Autodesk Inventor part; units mm, degrees
(part 2 of 2)
sketch "Эскиз21" plane through (0, 6, 0) normal (0, 1, 0) x (1, 0, 0)
  line L0 (0, 0) -> (0, 250) construction
  line L1 (140, 250) -> (-140, 250) construction
  line L2 (0, 125) -> (37.5, 125) construction
  line L3 (17.5, 87.5) -> (57.5, 87.5)
  line L4 (57.5, 87.5) -> (57.5, 162.5)
  line L5 (57.5, 162.5) -> (17.5, 162.5)
  line L6 (17.5, 162.5) -> (17.5, 87.5)
  line L7 (17.5, 87.5) -> (57.5, 162.5) construction
  line L8 (57.5, 87.5) -> (17.5, 162.5) construction
  line L9 (0, 0) -> (150, 0)
  line L10 (150, -240) -> (150, 240) projected
  line L11 (17.5, 87.5) -> (17.5, 112.5)
  line L12 (17.5, 112.5) -> (57.5, 112.5)
  line L13 (17.5, 112.5) -> (17.5, 162.5)
  line L14 (17.5, 137.5) -> (57.5, 137.5)
  line L15 (-57.5, 137.5) -> (-17.5, 137.5)
  line L16 (-17.5, 162.5) -> (-57.5, 162.5)
  line L17 (-57.5, 112.5) -> (-17.5, 112.5)
  line L18 (-57.5, 112.5) -> (-57.5, 162.5)
  line L19 (-75, 125) -> (-37.5, 125) construction
  line L20 (-17.5, 87.5) -> (-17.5, 162.5)
  line L21 (-57.5, 87.5) -> (-17.5, 87.5)
  line L22 (-57.5, 87.5) -> (-17.5, 162.5) construction
  line L23 (-57.5, 87.5) -> (-57.5, 112.5)
  line L24 (-57.5, 162.5) -> (-57.5, 87.5)
  line L25 (-17.5, 87.5) -> (-57.5, 162.5) construction
  line L26 (17.5, -112.5) -> (57.5, -112.5)
  line L27 (57.5, -87.5) -> (17.5, -87.5)
  line L28 (17.5, -137.5) -> (57.5, -137.5)
  line L29 (17.5, -137.5) -> (17.5, -87.5)
  line L30 (0, -125) -> (37.5, -125) construction
  line L31 (57.5, -162.5) -> (57.5, -87.5)
  line L32 (17.5, -162.5) -> (57.5, -162.5)
  line L33 (17.5, -162.5) -> (57.5, -87.5) construction
  line L34 (17.5, -162.5) -> (17.5, -137.5)
  line L35 (17.5, -87.5) -> (17.5, -162.5)
  line L36 (57.5, -162.5) -> (17.5, -87.5) construction
  line L37 (-57.5, -112.5) -> (-17.5, -112.5)
  line L38 (-17.5, -87.5) -> (-57.5, -87.5)
  line L39 (-57.5, -137.5) -> (-17.5, -137.5)
  line L40 (-57.5, -137.5) -> (-57.5, -87.5)
  line L41 (-75, -125) -> (-37.5, -125) construction
  line L42 (-17.5, -162.5) -> (-17.5, -87.5)
  line L43 (-57.5, -162.5) -> (-17.5, -162.5)
  line L44 (-57.5, -162.5) -> (-17.5, -87.5) construction
  line L45 (-57.5, -162.5) -> (-57.5, -137.5)
  line L46 (-57.5, -87.5) -> (-57.5, -162.5)
  line L47 (-17.5, -162.5) -> (-57.5, -87.5) construction
  dimension "d289" = 40
  dimension "d296" = 75
  dimension "d299" = 250
  constraints: 92 end point, 12 midpoint, 12 point on line, 3 horizontal, 3 perpendicular, 2 parallel, 1 collinear, 1 vertical, 63 other
  measures "d289" distance of L5.end L4.end
  measures "d296" distance of L4.end L16.start
  measures "d299" distance of L4.end L27.start
extrude "Выдавливание18" cut sketch "Эскиз21" against normal blind 6 contours L6 L5 L4 L14 | L18 L16 L20 L15 | L28 L31 L32 L34 | L39 L42 L43 L45 bodies 1
sketch "Эскиз22" plane through (3, 0, 108.75) normal (1, 0, 0) x (0, 0, -1)
  arc A0 (306.75, 506) -> (308.75, 508) centre (306.75, 508) ccw projected
  line L0 (308.75, 508) -> (308.75, 596) projected
  arc A1 (308.75, 596) -> (298.75, 606) centre (298.75, 596) ccw projected
  line L1 (298.75, 606) -> (111.75, 606) projected
  line L2 (111.75, 606) -> (111.75, 306) projected
  line L3 (111.75, 306) -> (105.75, 306) projected
  line L4 (105.75, 306) -> (105.75, 606) projected
  line L5 (105.75, 606) -> (-81.25, 606) projected
  arc A2 (-81.25, 606) -> (-91.25, 596) centre (-81.25, 596) ccw projected
  line L6 (-91.25, 596) -> (-91.25, 508) projected
  arc A3 (-91.25, 508) -> (-89.25, 506) centre (-89.25, 508) ccw projected
  line L7 (-89.25, 506) -> (-85.75, 506) projected
  arc A4 (-83.75, 504) -> (-85.75, 506) centre (-85.75, 504) ccw projected
  line L8 (-83.75, 504) -> (-83.75, 158) projected
  arc A5 (-85.75, 156) -> (-83.75, 158) centre (-85.75, 158) ccw projected
  line L9 (-85.75, 156) -> (-89.25, 156) projected
  arc A6 (-89.25, 156) -> (-91.25, 154) centre (-89.25, 154) ccw projected
  line L10 (-91.25, 154) -> (-91.25, 66) projected
  arc A7 (-101.25, 56) -> (-91.25, 66) centre (-101.25, 66) ccw projected
  line L11 (-101.25, 56) -> (-131.25, 56) projected
  arc A8 (-131.25, 56) -> (-141.25, 46) centre (-131.25, 46) ccw projected
  line L12 (-141.25, 46) -> (-141.25, 6) projected
  line L13 (-141.25, 6) -> (-125, 6) projected
  line L14 (-125, 6) -> (-125, 0) projected
  line L15 (-95, 0) -> (-125, 0) projected
  line L16 (-95, 6) -> (-95, 0) projected
  line L17 (-95, 6) -> (-80.75, 6) projected
  line L18 (-80.75, 6) -> (-80.75, 9) projected
  line L19 (-80.75, 9) -> (-82.15, 9) projected
  line L20 (-82.15, 9) -> (-82.15, 12.1) projected
  line L21 (-82.15, 12.1) -> (-80.75, 12.1) projected
  line L22 (-80.75, 12.1) -> (-80.75, 21) projected
  line L23 (-80.75, 21) -> (-76.75, 21) projected
  line L24 (-76.75, 21) -> (-76.75, 12.1) projected
  line L25 (-76.75, 12.1) -> (-75.35, 12.1) projected
  line L26 (-75.35, 12.1) -> (-75.35, 9) projected
  line L27 (-75.35, 9) -> (-76.75, 9) projected
  line L28 (-76.75, 9) -> (-76.75, 6) projected
  line L29 (-76.75, 6) -> (-62.5, 6) projected
  line L30 (-62.5, 6) -> (-62.5, 0) projected
  line L31 (-32.5, 0) -> (-62.5, 0) projected
  line L32 (-32.5, 6) -> (-32.5, 0) projected
  line L33 (-32.5, 6) -> (0, 6) projected
  line L34 (0, 6) -> (0, 0) projected
  line L35 (30, 0) -> (0, 0) projected
  line L36 (30, 6) -> (30, 0) projected
  line L37 (30, 6) -> (44.25, 6) projected
  line L38 (44.25, 6) -> (44.25, 9) projected
  line L39 (44.25, 9) -> (42.83, 9) projected
  line L40 (42.83, 9) -> (42.83, 12.1) projected
  line L41 (42.83, 12.1) -> (44.25, 12.1) projected
  line L42 (44.25, 12.1) -> (44.25, 21) projected
  line L43 (44.25, 21) -> (48.25, 21) projected
  line L44 (48.25, 21) -> (48.25, 12.1) projected
  line L45 (48.25, 12.1) -> (49.67, 12.1) projected
  line L46 (49.67, 12.1) -> (49.67, 9) projected
  line L47 (49.67, 9) -> (48.25, 9) projected
  line L48 (48.25, 9) -> (48.25, 6) projected
  line L49 (48.25, 6) -> (62.5, 6) projected
  line L50 (62.5, 6) -> (62.5, 0) projected
  line L51 (92.5, 0) -> (62.5, 0) projected
  line L52 (92.5, 6) -> (92.5, 0) projected
  line L53 (92.5, 6) -> (125, 6) projected
  line L54 (125, 6) -> (125, 0) projected
  line L55 (155, 0) -> (125, 0) projected
  line L56 (155, 6) -> (155, 0) projected
  line L57 (155, 6) -> (169.25, 6) projected
  line L58 (169.25, 6) -> (169.25, 9) projected
  line L59 (169.25, 9) -> (167.83, 9) projected
  line L60 (167.83, 9) -> (167.83, 12.1) projected
  line L61 (167.83, 12.1) -> (169.25, 12.1) projected
  line L62 (169.25, 12.1) -> (169.25, 21) projected
  line L63 (169.25, 21) -> (173.25, 21) projected
  line L64 (173.25, 21) -> (173.25, 12.1) projected
  line L65 (173.25, 12.1) -> (174.67, 12.1) projected
  line L66 (174.67, 12.1) -> (174.67, 9) projected
  line L67 (174.67, 9) -> (173.25, 9) projected
  line L68 (173.25, 9) -> (173.25, 6) projected
  line L69 (173.25, 6) -> (187.5, 6) projected
  line L70 (187.5, 6) -> (187.5, 0) projected
  line L71 (217.5, 0) -> (187.5, 0) projected
  line L72 (217.5, 6) -> (217.5, 0) projected
  line L73 (217.5, 6) -> (250, 6) projected
  line L74 (250, 6) -> (250, 0) projected
  line L75 (280, 0) -> (250, 0) projected
  line L76 (280, 6) -> (280, 0) projected
  line L77 (280, 6) -> (294.25, 6) projected
  line L78 (294.25, 6) -> (294.25, 9) projected
  line L79 (294.25, 9) -> (292.83, 9) projected
  line L80 (292.83, 9) -> (292.83, 12.1) projected
  line L81 (292.83, 12.1) -> (294.25, 12.1) projected
  line L82 (294.25, 12.1) -> (294.25, 21) projected
  line L83 (294.25, 21) -> (298.25, 21) projected
  line L84 (298.25, 21) -> (298.25, 12.1) projected
  line L85 (298.25, 12.1) -> (299.67, 12.1) projected
  line L86 (299.67, 12.1) -> (299.67, 9) projected
  line L87 (299.67, 9) -> (298.25, 9) projected
  line L88 (298.25, 9) -> (298.25, 6) projected
  line L89 (298.25, 6) -> (312.5, 6) projected
  line L90 (312.5, 6) -> (312.5, 0) projected
  line L91 (342.5, 0) -> (312.5, 0) projected
  line L92 (342.5, 6) -> (342.5, 0) projected
  line L93 (342.5, 6) -> (358.75, 6) projected
  line L94 (358.75, 6) -> (358.75, 46) projected
  arc A9 (358.75, 46) -> (348.75, 56) centre (348.75, 46) ccw projected
  line L95 (348.75, 56) -> (318.75, 56) projected
  arc A10 (308.75, 66) -> (318.75, 56) centre (318.75, 66) ccw projected
  line L96 (308.75, 66) -> (308.75, 154) projected
  arc A11 (308.75, 154) -> (306.75, 156) centre (306.75, 154) ccw projected
  line L97 (306.75, 156) -> (303.25, 156) projected
  arc A12 (301.25, 158) -> (303.25, 156) centre (303.25, 158) ccw projected
  line L98 (301.25, 158) -> (301.25, 504) projected
  arc A13 (303.25, 506) -> (301.25, 504) centre (303.25, 504) ccw projected
  line L99 (303.25, 506) -> (306.75, 506) projected
  circle A14 centre (126.25, 583.5) radius 2 projected
  circle A15 centre (71.25, 583.5) radius 2 projected
  circle A16 centre (146.25, 583.5) radius 2 projected
  circle A17 centre (91.25, 583.5) radius 2 projected
  line L100 (198.75, 456) -> (268.75, 456) projected
  arc A18 (268.75, 446) -> (268.75, 456) centre (268.75, 451) ccw projected
  line L101 (268.75, 446) -> (198.75, 446) projected
  arc A19 (198.75, 456) -> (198.75, 446) centre (198.75, 451) ccw projected
  line L102 (198.75, 286) -> (268.75, 286) projected
  arc A20 (268.75, 276) -> (268.75, 286) centre (268.75, 281) ccw projected
  line L103 (268.75, 276) -> (198.75, 276) projected
  arc A21 (198.75, 286) -> (198.75, 276) centre (198.75, 281) ccw projected
  line L104 (-51.25, 456) -> (18.75, 456) projected
  arc A22 (18.75, 446) -> (18.75, 456) centre (18.75, 451) ccw projected
  line L105 (18.75, 446) -> (-51.25, 446) projected
  arc A23 (-51.25, 456) -> (-51.25, 446) centre (-51.25, 451) ccw projected
  line L106 (-51.25, 286) -> (18.75, 286) projected
  arc A24 (18.75, 276) -> (18.75, 286) centre (18.75, 281) ccw projected
  line L107 (18.75, 276) -> (-51.25, 276) projected
  arc A25 (-51.25, 286) -> (-51.25, 276) centre (-51.25, 281) ccw projected
  line L108 (-51.25, 116) -> (18.75, 116) projected
  arc A26 (18.75, 106) -> (18.75, 116) centre (18.75, 111) ccw projected
  line L109 (18.75, 106) -> (-51.25, 106) projected
  arc A27 (-51.25, 116) -> (-51.25, 106) centre (-51.25, 111) ccw projected
  line L110 (-51.25, 201) -> (18.75, 201) projected
  arc A28 (18.75, 191) -> (18.75, 201) centre (18.75, 196) ccw projected
  line L111 (18.75, 191) -> (-51.25, 191) projected
  arc A29 (-51.25, 201) -> (-51.25, 191) centre (-51.25, 196) ccw projected
  line L112 (-51.25, 371) -> (18.75, 371) projected
  arc A30 (18.75, 361) -> (18.75, 371) centre (18.75, 366) ccw projected
  line L113 (18.75, 361) -> (-51.25, 361) projected
  arc A31 (-51.25, 371) -> (-51.25, 361) centre (-51.25, 366) ccw projected
  line L114 (198.75, 201) -> (268.75, 201) projected
  arc A32 (268.75, 191) -> (268.75, 201) centre (268.75, 196) ccw projected
  line L115 (268.75, 191) -> (198.75, 191) projected
  arc A33 (198.75, 201) -> (198.75, 191) centre (198.75, 196) ccw projected
  line L116 (198.75, 371) -> (268.75, 371) projected
  arc A34 (268.75, 361) -> (268.75, 371) centre (268.75, 366) ccw projected
  line L117 (268.75, 361) -> (198.75, 361) projected
  arc A35 (198.75, 371) -> (198.75, 361) centre (198.75, 366) ccw projected
  line L118 (198.75, 116) -> (268.75, 116) projected
  arc A36 (268.75, 106) -> (268.75, 116) centre (268.75, 111) ccw projected
  line L119 (268.75, 106) -> (198.75, 106) projected
  arc A37 (198.75, 116) -> (198.75, 106) centre (198.75, 111) ccw projected
  line L120 (-91.25, 508) -> (-91.25, 596) projected
  line L121 (-91.25, 599) -> (-82.25, 599) construction
  line L122 (-81.25, 606) -> (105.75, 606) projected
  line L123 (-82.25, 606) -> (-82.25, 599) construction
  circle A38 centre (-82.25, 599) radius 2.1
  line L124 (-82.25, 599) -> (-71.25, 599) construction
  circle A39 centre (-71.25, 599) radius 2.1
  line L125 (-91.25, 556) -> (-44.3375, 556) construction
  circle A40 centre (-38.25, 585) radius 2.1
  line L126 (-38.25, 585) -> (-38.25, 556) construction
  line L127 (-91.25, 513) -> (-82.25, 513) construction
  line L128 (-82.25, 506) -> (-82.25, 513) construction
  circle A41 centre (-82.25, 513) radius 2.1
  line L129 (-82.25, 513) -> (-71.25, 513) construction
  circle A42 centre (-71.25, 513) radius 2.1
  circle A43 centre (-38.25, 527) radius 2.1
  line L130 (-16.25, 571.25) -> (35.603, 571.25) construction
  line L131 (18.55, 571.25) -> (18.55, 597.185) construction
  circle A44 centre (18.55, 597.185) radius 2.1
  circle A45 centre (-1.45, 597.185) radius 2.1
  circle A46 centre (-21.45, 597.185) radius 2.1
  circle A47 centre (18.55, 545.315) radius 2.1
  circle A48 centre (-1.45, 545.315) radius 2.1
  circle A49 centre (-21.45, 545.315) radius 2.1
  line L132 (108.75, 616.4203) -> (108.75, 456.3683) construction
  line L133 (111.75, 368.404) -> (111.75, 606) projected
  line L134 (108.75, 537.7397) -> (308.75, 537.7397) construction
  line L135 (108.75, 537.7397) -> (-91.25, 537.7397) construction
  line L136 (308.75, 508) -> (308.75, 596)
  line L137 (308.75, 599) -> (299.75, 599) construction
  line L138 (299.75, 606) -> (299.75, 599) construction
  circle A50 centre (299.75, 599) radius 2.1
  line L139 (299.75, 599) -> (288.75, 599) construction
  circle A51 centre (288.75, 599) radius 2.1
  circle A52 centre (255.75, 585) radius 2.1
  circle A53 centre (255.75, 527) radius 2.1
  circle A54 centre (288.75, 513) radius 2.1
  circle A55 centre (299.75, 513) radius 2.1
  circle A56 centre (198.95, 597.185) radius 2.1
  circle A57 centre (218.95, 597.185) radius 2.1
  circle A58 centre (238.95, 597.185) radius 2.1
  circle A59 centre (198.95, 545.315) radius 2.1
  circle A60 centre (218.95, 545.315) radius 2.1
  circle A61 centre (238.95, 545.315) radius 2.1
  point P0 (108.75, 0)
  dimension "d302" = 9
  dimension "d303" = 7
  dimension "d304" = 4.2
  dimension "d305" = 11
  dimension "d306" = 43
  dimension "d307" = 29
  dimension "d308" = 53
  dimension "d309" = 34.75
  dimension "d310" = 25.935
  dimension "d313" = 20
  dimension "d316" = 51.87
  dimension "d319" = 16.8
  constraints: 34 end point, 26 symmetric about line, 24 centre point, 10 coincident, 10 point on line, 5 perpendicular, 4 horizontal, 3 equal radius, 1 collinear, 1 parallel, 1 vertical, 25 other
  measures "d302" distance of L121.start L121.end
  measures "d303" distance of L123.start L121.end
  measures "d304" diameter of A38
  measures "d305" distance of L124.start L124.end
  measures "d306" distance between parallel lines of L121 L125
  measures "d307" distance of L126.start L126.end
  measures "d308" distance between parallel lines of L6 L126
  measures "d309" distance between parallel lines of L130 L5
  measures "d310" distance of L131.start L131.end
  measures "d313" distance of A44.centre A45.centre
  measures "d316" distance of A44.centre A47.centre
  measures "d319" distance from line of L126 A46.centre
extrude "Выдавливание19" cut sketch "Эскиз22" against normal blind 10 contours A14 | A15 | A16 | A17 | L100 A18 L101 A19 | L104 A22 L105 A23 | A38 | A39 | A40 | A41 | A42 | A43 | A44 | A45 | A46 | A47 | A48 | A49 | A50 | A51 | A52 | A53 | A54 | A55 | A56 | A57 | A58 | A59 | A60 | A61 bodies 2
